Autodesk Fusion 360 part; units mm, degrees
note: some values were not read from the file. Set by a fixed rule: which face or edge a step refers to.
(part 8 of 20)
  spline S44 degree 5 poles (-3.681, 14.0486) (-3.681, 14.0487) (-3.681, 14.0488) (-3.6811, 14.0491) (-3.6812, 14.0494) (-3.6813, 14.0499) (-3.6815, 14.0505) (-3.6817, 14.0512) (-3.6819, 14.0519) (-3.6821, 14.0528) (-3.6824, 14.0537) (-3.6827, 14.0546) (-3.683, 14.0557) (-3.6833, 14.0568) (-3.6837, 14.058) (-3.6841, 14.0592) (-3.6845, 14.0606) (-3.6849, 14.0619) (-3.6853, 14.0634) (-3.6858, 14.0649) (-3.6863, 14.0665) (-3.6869, 14.0682) (-3.6874, 14.0699) (-3.688, 14.0717) (-3.6886, 14.0736) (-3.6892, 14.0755) (-3.6899, 14.0775) (-3.6906, 14.0795) (-3.6913, 14.0816) (-3.692, 14.0838) (-3.6928, 14.086) (-3.6936, 14.0883) (-3.6944, 14.0906) (-3.6952, 14.093) (-3.6961, 14.0955) (-3.697, 14.098) (-3.6979, 14.1006) (-3.6988, 14.1032) (-3.6998, 14.1059) (-3.7008, 14.1086) (-3.7018, 14.1114) (-3.7029, 14.1143) (-3.704, 14.1172) (-3.7051, 14.1202) (-3.7062, 14.1232) (-3.7073, 14.1262) (-3.7085, 14.1293) (-3.7097, 14.1325) (-3.711, 14.1357) (-3.7123, 14.139) (-3.7136, 14.1423) (-3.7149, 14.1457) (-3.7162, 14.1491) (-3.7176, 14.1525) (-3.719, 14.1561) (-3.7204, 14.1596) (-3.7219, 14.1632) (-3.7234, 14.1669) (-3.7249, 14.1706) (-3.7265, 14.1743) (-3.728, 14.1781) (-3.7296, 14.1819) (-3.7313, 14.1858) (-3.7329, 14.1898) (-3.7346, 14.1937) (-3.7363, 14.1977) (-3.7381, 14.2018) (-3.7398, 14.2059) (-3.7416, 14.21) (-3.7435, 14.2142) (-3.7453, 14.2185) (-3.7472, 14.2227) (-3.7491, 14.227) (-3.7511, 14.2314) (-3.753, 14.2358) (-3.755, 14.2402) (-3.7571, 14.2447) (-3.7591, 14.2492) (-3.7612, 14.2537) (-3.7633, 14.2583) (-3.7655, 14.263) (-3.7676, 14.2676) (-3.7698, 14.2723) (-3.7721, 14.2771) (-3.7743, 14.2819) (-3.7766, 14.2867) (-3.7789, 14.2915) (-3.7813, 14.2964) (-3.7836, 14.3013) (-3.7861, 14.3063) (-3.7885, 14.3113) (-3.791, 14.3163) (-3.7934, 14.3214) (-3.796, 14.3265) (-3.7985, 14.3316) (-3.8011, 14.3368) (-3.8037, 14.342) (-3.8063, 14.3473) (-3.809, 14.3525) (-3.8117, 14.3578) (-3.8144, 14.3632) (-3.8172, 14.3685) (-3.82, 14.3739) (-3.8228, 14.3794) (-3.8257, 14.3848) (-3.8285, 14.3903) (-3.8314, 14.3959) (-3.8344, 14.4014) (-3.8373, 14.407) (-3.8403, 14.4126) (-3.8434, 14.4183) (-3.8464, 14.424) (-3.8495, 14.4297) (-3.8526, 14.4354) (-3.8558, 14.4412) (-3.8589, 14.447) (-3.8621, 14.4528) (-3.8654, 14.4587) (-3.8686, 14.4645) (-3.8719, 14.4704) (-3.8752, 14.4764) (-3.8786, 14.4824) (-3.882, 14.4883) (-3.8854, 14.4944) (-3.8888, 14.5004) (-3.8923, 14.5065) (-3.8958, 14.5126) (-3.8993, 14.5187) (-3.9029, 14.5249) (-3.9065, 14.5311) (-3.9101, 14.5373) (-3.9138, 14.5435) (-3.9175, 14.5497) (-3.9212, 14.556) (-3.9249, 14.5623) (-3.9287, 14.5687) (-3.9325, 14.575) (-3.9363, 14.5814) (-3.9402, 14.5878) (-3.9441, 14.5942) (-3.948, 14.6007) (-3.952, 14.6072) (-3.9559, 14.6137) (-3.96, 14.6202) (-3.964, 14.6267) (-3.9681, 14.6333) (-3.9722, 14.6399) (-3.9763, 14.6465) (-3.9805, 14.6531) (-3.9847, 14.6598) (-3.9889, 14.6665) (-3.9932, 14.6731) (-3.9974, 14.6799) (-4.0018, 14.6866) (-4.0061, 14.6934) (-4.0105, 14.7002) (-4.0149, 14.707) (-4.0193, 14.7138) (-4.0238, 14.7206) (-4.0283, 14.7275) (-4.0328, 14.7344) (-4.0374, 14.7413) (-4.042, 14.7482) (-4.0466, 14.7551) (-4.0512, 14.7621) (-4.0559, 14.7691) (-4.0606, 14.7761) (-4.0654, 14.7831) (-4.0701, 14.7901) (-4.0749, 14.7972) (-4.0798, 14.8043) (-4.0846, 14.8114) (-4.0895, 14.8185) (-4.0944, 14.8256) (-4.0994, 14.8328) (-4.1044, 14.8399) (-4.1094, 14.8471) (-4.1144, 14.8543) (-4.1195, 14.8615) (-4.1246, 14.8687) (-4.1297, 14.876) (-4.1349, 14.8833) (-4.1401, 14.8905) (-4.1453, 14.8978) (-4.1506, 14.9052) (-4.1559, 14.9125) (-4.1612, 14.9198) (-4.1665, 14.9272) (-4.1719, 14.9346) (-4.1773, 14.942) (-4.1827, 14.9494) (-4.1882, 14.9568) (-4.1937, 14.9642) (-4.1992, 14.9717) (-4.2048, 14.9791) (-4.2104, 14.9866) (-4.216, 14.9941) (-4.2216, 15.0016) (-4.2273, 15.0092) (-4.233, 15.0167) (-4.2388, 15.0242) (-4.2445, 15.0318) (-4.2503, 15.0394) (-4.2562, 15.047) (-4.262, 15.0546) (-4.2679, 15.0622) (-4.2738, 15.0698) (-4.2798, 15.0775) (-4.2858, 15.0851) (-4.2918, 15.0928) (-4.2978, 15.1005) (-4.3039, 15.1082) (-4.31, 15.1159) (-4.3161, 15.1236) (-4.3223, 15.1313) (-4.3285, 15.1391) (-4.3347, 15.1468) (-4.3409, 15.1546) (-4.3472, 15.1624) (-4.3535, 15.1702) (-4.3599, 15.178) (-4.3662, 15.1858) (-4.3726, 15.1936) (-4.3791, 15.2014) (-4.3855, 15.2093) (-4.392, 15.2171) (-4.3985, 15.225) (-4.4051, 15.2329) (-4.4117, 15.2407) (-4.4183, 15.2486) (-4.4249, 15.2565) (-4.4316, 15.2645) (-4.4383, 15.2724) (-4.445, 15.2803) (-4.4518, 15.2883) (-4.4586, 15.2962) (-4.4654, 15.3042) (-4.4722, 15.3121) (-4.4791, 15.3201) (-4.486, 15.3281) (-4.493, 15.3361) (-4.4985, 15.3425) (-4.5027, 15.3473) (-4.5055, 15.3505) (-4.5069, 15.3521) knots 0 0 0 0 0 0 0.00416667 0.00833333 0.0125 0.01666667 0.02083333 0.025 0.02916667 0.03333333 0.0375 0.04166667 0.04583333 0.05 0.05416667 0.05833333 0.0625 0.06666667 0.07083333 0.075 0.07916667 0.08333333 0.0875 0.09166667 0.09583333 0.1 0.10416667 0.10833333 0.1125 0.11666667 0.12083333 0.125 0.12916667 0.13333333 0.1375 0.14166667 0.14583333 0.15 0.15416667 0.15833333 0.1625 0.16666667 0.17083333 0.175 0.17916667 0.18333333 0.1875 0.19166667 0.19583333 0.2 0.20416667 0.20833333 0.2125 0.21666667 0.22083333 0.225 0.22916667 0.23333333 0.2375 0.24166667 0.24583333 0.25 0.25416667 0.25833333 0.2625 0.26666667 0.27083333 0.275 0.27916667 0.28333333 0.2875 0.29166667 0.29583333 0.3 0.30416667 0.30833333 0.3125 0.31666667 0.32083333 0.325 0.32916667 0.33333333 0.3375 0.34166667 0.34583333 0.35 0.35416667 0.35833333 0.3625 0.36666667 0.37083333 0.375 0.37916667 0.38333333 0.3875 0.39166667 0.39583333 0.4 0.40416667 0.40833333 0.4125 0.41666667 0.42083333 0.425 0.42916667 0.43333333 0.4375 0.44166667 0.44583333 0.45 0.45416667 0.45833333 0.4625 0.46666667 0.47083333 0.475 0.47916667 0.48333333 0.4875 0.49166667 0.49583333 0.5 0.50416667 0.50833333 0.5125 0.51666667 0.52083333 0.525 0.52916667 0.53333333 0.5375 0.54166667 0.54583333 0.55 0.55416667 0.55833333 0.5625 0.56666667 0.57083333 0.575 0.57916667 0.58333333 0.5875 0.59166667 0.59583333 0.6 0.60416667 0.60833333 0.6125 0.61666667 0.62083333 0.625 0.62916667 0.63333333 0.6375 0.64166667 0.64583333 0.65 0.65416667 0.65833333 0.6625 0.66666667 0.67083333 0.675 0.67916667 0.68333333 0.6875 0.69166667 0.69583333 0.7 0.70416667 0.70833333 0.7125 0.71666667 0.72083333 0.725 0.72916667 0.73333333 0.7375 0.74166667 0.74583333 0.75 0.75416667 0.75833333 0.7625 0.76666667 0.77083333 0.775 0.77916667 0.78333333 0.7875 0.79166667 0.79583333 0.8 0.80416667 0.80833333 0.8125 0.81666667 0.82083333 0.825 0.82916667 0.83333333 0.8375 0.84166667 0.84583333 0.85 0.85416667 0.85833333 0.8625 0.86666667 0.87083333 0.875 0.87916667 0.88333333 0.8875 0.89166667 0.89583333 0.9 0.90416667 0.90833333 0.9125 0.91666667 0.92083333 0.925 0.92916667 0.93333333 0.9375 0.94166667 0.94583333 0.95 0.95416667 0.95833333 0.9625 0.96666667 0.97083333 0.975 0.97916667 0.98333333 0.9875 0.99166667 0.99583333 1 1 1 1 1 1
  spline S45 degree 5 poles (-12.6699, -9.771) (-12.6679, -9.7705) (-12.6637, -9.7696) (-12.6575, -9.7682) (-12.6492, -9.7663) (-12.6389, -9.7639) (-12.6286, -9.7615) (-12.6184, -9.7591) (-12.6081, -9.7566) (-12.5979, -9.7542) (-12.5878, -9.7518) (-12.5776, -9.7493) (-12.5675, -9.7469) (-12.5574, -9.7444) (-12.5474, -9.7419) (-12.5374, -9.7394) (-12.5274, -9.7369) (-12.5174, -9.7344) (-12.5075, -9.7319) (-12.4976, -9.7293) (-12.4877, -9.7268) (-12.4779, -9.7243) (-12.4681, -9.7217) (-12.4583, -9.7191) (-12.4486, -9.7166) (-12.4389, -9.714) (-12.4292, -9.7114) (-12.4195, -9.7088) (-12.4099, -9.7062) (-12.4003, -9.7036) (-12.3908, -9.7009) (-12.3812, -9.6983) (-12.3717, -9.6957) (-12.3623, -9.693) (-12.3528, -9.6904) (-12.3434, -9.6877) (-12.3341, -9.685) (-12.3247, -9.6823) (-12.3154, -9.6797) (-12.3062, -9.677) (-12.2969, -9.6743) (-12.2877, -9.6716) (-12.2785, -9.6688) (-12.2694, -9.6661) (-12.2603, -9.6634) (-12.2512, -9.6607) (-12.2421, -9.6579) (-12.2331, -9.6552) (-12.2241, -9.6524) (-12.2152, -9.6496) (-12.2063, -9.6469) (-12.1974, -9.6441) (-12.1885, -9.6413) (-12.1797, -9.6385) (-12.1709, -9.6357) (-12.1622, -9.6329) (-12.1535, -9.6301) (-12.1448, -9.6273) (-12.1361, -9.6245) (-12.1275, -9.6217) (-12.1189, -9.6189) (-12.1104, -9.616) (-12.1018, -9.6132) (-12.0934, -9.6104) (-12.0849, -9.6075) (-12.0765, -9.6047) (-12.0681, -9.6018) (-12.0598, -9.599) (-12.0515, -9.5961) (-12.0432, -9.5933) (-12.035, -9.5904) (-12.0267, -9.5875) (-12.0186, -9.5846) (-12.0104, -9.5818) (-12.0023, -9.5789) (-11.9943, -9.576) (-11.9862, -9.5731) (-11.9782, -9.5702) (-11.9703, -9.5673) (-11.9624, -9.5644) (-11.9545, -9.5615) (-11.9466, -9.5586) (-11.9388, -9.5557) (-11.931, -9.5528) (-11.9233, -9.5499) (-11.9156, -9.547) (-11.9079, -9.5441) (-11.9002, -9.5412) (-11.8926, -9.5383) (-11.8851, -9.5354) (-11.8776, -9.5325) (-11.8701, -9.5295) (-11.8626, -9.5266) (-11.8552, -9.5237) (-11.8478, -9.5208) (-11.8405, -9.5179) (-11.8332, -9.515) (-11.8259, -9.512) (-11.8187, -9.5091) (-11.8115, -9.5062) (-11.8043, -9.5033) (-11.7972, -9.5004) (-11.7901, -9.4975) (-11.7831, -9.4945) (-11.7761, -9.4916) (-11.7691, -9.4887) (-11.7622, -9.4858) (-11.7553, -9.4829) (-11.7484, -9.48) (-11.7416, -9.4771) (-11.7348, -9.4742) (-11.7281, -9.4713) (-11.7214, -9.4684) (-11.7148, -9.4655) (-11.7081, -9.4626) (-11.7016, -9.4597) (-11.695, -9.4568) (-11.6885, -9.4539) (-11.6821, -9.451) (-11.6756, -9.4482) (-11.6693, -9.4453) (-11.6629, -9.4424) (-11.6566, -9.4396) (-11.6504, -9.4367) (-11.6441, -9.4338) (-11.638, -9.431) (-11.6318, -9.4281) (-11.6257, -9.4253) (-11.6197, -9.4225) (-11.6137, -9.4196) (-11.6077, -9.4168) (-11.6017, -9.414) (-11.5959, -9.4112) (-11.59, -9.4084) (-11.5842, -9.4056) (-11.5784, -9.4028) (-11.5727, -9.4) (-11.567, -9.3972) (-11.5614, -9.3944) (-11.5558, -9.3917) (-11.5502, -9.3889) (-11.5447, -9.3862) (-11.5392, -9.3834) (-11.5338, -9.3807) (-11.5284, -9.378) (-11.5231, -9.3753) (-11.5178, -9.3725) (-11.5125, -9.3699) (-11.5073, -9.3672) (-11.5021, -9.3645) (-11.497, -9.3618) (-11.4919, -9.3592) (-11.4869, -9.3565) (-11.4819, -9.3539) (-11.4769, -9.3513) (-11.472, -9.3487) (-11.4672, -9.3461) (-11.4623, -9.3435) (-11.4576, -9.3409) (-11.4528, -9.3383) (-11.4482, -9.3358) (-11.4435, -9.3332) (-11.4389, -9.3307) (-11.4344, -9.3282) (-11.4299, -9.3257) (-11.4254, -9.3232) (-11.421, -9.3207) (-11.4167, -9.3183) (-11.4123, -9.3158) (-11.4081, -9.3134) (-11.4038, -9.311) (-11.3997, -9.3086) (-11.3955, -9.3062) (-11.3915, -9.3039) (-11.3874, -9.3015) (-11.3834, -9.2992) (-11.3795, -9.2969) (-11.3756, -9.2946) (-11.3718, -9.2923) (-11.368, -9.2901) (-11.3642, -9.2878) (-11.3605, -9.2856) (-11.3569, -9.2834) (-11.3533, -9.2812) (-11.3497, -9.2791) (-11.3462, -9.2769) (-11.3428, -9.2748) (-11.3394, -9.2727) (-11.336, -9.2706) (-11.3327, -9.2685) (-11.3295, -9.2665) (-11.3263, -9.2645) (-11.3231, -9.2625) (-11.32, -9.2605) (-11.317, -9.2586) (-11.314, -9.2567) (-11.311, -9.2548) (-11.3081, -9.2529) (-11.3053, -9.2511) (-11.3025, -9.2492) (-11.2998, -9.2474) (-11.2971, -9.2457) (-11.2944, -9.2439) (-11.2919, -9.2422) (-11.2893, -9.2405) (-11.2869, -9.2389) (-11.2844, -9.2372) (-11.2821, -9.2356) (-11.2798, -9.2341) (-11.2775, -9.2325) (-11.2753, -9.231) (-11.2732, -9.2295) (-11.2711, -9.2281) (-11.269, -9.2266) (-11.2671, -9.2253) (-11.2651, -9.2239) (-11.2633, -9.2226) (-11.2615, -9.2213) (-11.2597, -9.22) (-11.258, -9.2188) (-11.2564, -9.2177) (-11.2548, -9.2165) (-11.2533, -9.2154) (-11.2518, -9.2143) (-11.2504, -9.2133) (-11.2491, -9.2123) (-11.2478, -9.2113) (-11.2465, -9.2104) (-11.2454, -9.2096) (-11.2443, -9.2087) (-11.2432, -9.2079) (-11.2422, -9.2072) (-11.2413, -9.2065) (-11.2404, -9.2058) (-11.2396, -9.2052) (-11.2389, -9.2046) (-11.2382, -9.2041) (-11.2376, -9.2036) (-11.2371, -9.2032) (-11.2366, -9.2028) (-11.2362, -9.2025) (-11.2359, -9.2022) (-11.2357, -9.2021) (-11.2356, -9.202) (-11.2355, -9.202) knots -1 -1 -1 -1 -1 -1 -0.99583333 -0.99166667 -0.9875 -0.98333333 -0.97916667 -0.975 -0.97083333 -0.96666667 -0.9625 -0.95833333 -0.95416667 -0.95 -0.94583333 -0.94166667 -0.9375 -0.93333333 -0.92916667 -0.925 -0.92083333 -0.91666667 -0.9125 -0.90833333 -0.90416667 -0.9 -0.89583333 -0.89166667 -0.8875 -0.88333333 -0.87916667 -0.875 -0.87083333 -0.86666667 -0.8625 -0.85833333 -0.85416667 -0.85 -0.84583333 -0.84166667 -0.8375 -0.83333333 -0.82916667 -0.825 -0.82083333 -0.81666667 -0.8125 -0.80833333 -0.80416667 -0.8 -0.79583333 -0.79166667 -0.7875 -0.78333333 -0.77916667 -0.775 -0.77083333 -0.76666667 -0.7625 -0.75833333 -0.75416667 -0.75 -0.74583333 -0.74166667 -0.7375 -0.73333333 -0.72916667 -0.725 -0.72083333 -0.71666667 -0.7125 -0.70833333 -0.70416667 -0.7 -0.69583333 -0.69166667 -0.6875 -0.68333333 -0.67916667 -0.675 -0.67083333 -0.66666667 -0.6625 -0.65833333 -0.65416667 -0.65 -0.64583333 -0.64166667 -0.6375 -0.63333333 -0.62916667 -0.625 -0.62083333 -0.61666667 -0.6125 -0.60833333 -0.60416667 -0.6 -0.59583333 -0.59166667 -0.5875 -0.58333333 -0.57916667 -0.575 -0.57083333 -0.56666667 -0.5625 -0.55833333 -0.55416667 -0.55 -0.54583333 -0.54166667 -0.5375 -0.53333333 -0.52916667 -0.525 -0.52083333 -0.51666667 -0.5125 -0.50833333 -0.50416667 -0.5 -0.49583333 -0.49166667 -0.4875 -0.48333333 -0.47916667 -0.475 -0.47083333 -0.46666667 -0.4625 -0.45833333 -0.45416667 -0.45 -0.44583333 -0.44166667 -0.4375 -0.43333333 -0.42916667 -0.425 -0.42083333 -0.41666667 -0.4125 -0.40833333 -0.40416667 -0.4 -0.39583333 -0.39166667 -0.3875 -0.38333333 -0.37916667 -0.375 -0.37083333 -0.36666667 -0.3625 -0.35833333 -0.35416667 -0.35 -0.34583333 -0.34166667 -0.3375 -0.33333333 -0.32916667 -0.325 -0.32083333 -0.31666667 -0.3125 -0.30833333 -0.30416667 -0.3 -0.29583333 -0.29166667 -0.2875 -0.28333333 -0.27916667 -0.275 -0.27083333 -0.26666667 -0.2625 -0.25833333 -0.25416667 -0.25 -0.24583333 -0.24166667 -0.2375 -0.23333333 -0.22916667 -0.225 -0.22083333 -0.21666667 -0.2125 -0.20833333 -0.20416667 -0.2 -0.19583333 -0.19166667 -0.1875 -0.18333333 -0.17916667 -0.175 -0.17083333 -0.16666667 -0.1625 -0.15833333 -0.15416667 -0.15 -0.14583333 -0.14166667 -0.1375 -0.13333333 -0.12916667 -0.125 -0.12083333 -0.11666667 -0.1125 -0.10833333 -0.10416667 -0.1 -0.09583333 -0.09166667 -0.0875 -0.08333333 -0.07916667 -0.075 -0.07083333 -0.06666667 -0.0625 -0.05833333 -0.05416667 -0.05 -0.04583333 -0.04166667 -0.0375 -0.03333333 -0.02916667 -0.025 -0.02083333 -0.01666667 -0.0125 -0.00833333 -0.00416667 0 0 0 0 0 0
  line L87 (-3.6808, 14.048) -> (-3.681, 14.0486)
  line L88 (-2.3514, 14.3312) -> (-2.3513, 14.3306)
  spline S46 degree 5 poles (-10.326, -10.2121) (-10.326, -10.2122) (-10.3261, -10.2123) (-10.3263, -10.2124) (-10.3266, -10.2127) (-10.3269, -10.2131) (-10.3274, -10.2135) (-10.3279, -10.214) (-10.3284, -10.2146) (-10.329, -10.2152) (-10.3296, -10.2159) (-10.3303, -10.2166) (-10.3311, -10.2174) (-10.3319, -10.2182) (-10.3327, -10.2191) (-10.3336, -10.2201) (-10.3346, -10.2211) (-10.3356, -10.2222) (-10.3366, -10.2233) (-10.3377, -10.2245) (-10.3388, -10.2257) (-10.34, -10.227) (-10.3412, -10.2284) (-10.3425, -10.2298) (-10.3438, -10.2312) (-10.3451, -10.2327) (-10.3465, -10.2343) (-10.3479, -10.2359) (-10.3494, -10.2376) (-10.3509, -10.2393) (-10.3525, -10.241) (-10.354, -10.2429) (-10.3557, -10.2447) (-10.3573, -10.2467) (-10.359, -10.2486) (-10.3608, -10.2507) (-10.3625, -10.2528) (-10.3643, -10.2549) (-10.3662, -10.2571) (-10.368, -10.2593) (-10.37, -10.2616) (-10.3719, -10.2639) (-10.3739, -10.2663) (-10.3759, -10.2688) (-10.3779, -10.2712) (-10.38, -10.2738) (-10.3821, -10.2764) (-10.3842, -10.279) (-10.3864, -10.2817) (-10.3886, -10.2844) (-10.3908, -10.2872) (-10.3931, -10.29) (-10.3954, -10.2929) (-10.3977, -10.2958) (-10.4, -10.2988) (-10.4024, -10.3018) (-10.4048, -10.3049) (-10.4072, -10.308) (-10.4096, -10.3112) (-10.4121, -10.3144) (-10.4146, -10.3176) (-10.4171, -10.3209) (-10.4197, -10.3243) (-10.4222, -10.3277) (-10.4248, -10.3311) (-10.4274, -10.3346) (-10.4301, -10.3382) (-10.4328, -10.3417) (-10.4354, -10.3454) (-10.4382, -10.349) (-10.4409, -10.3528) (-10.4436, -10.3565) (-10.4464, -10.3603) (-10.4492, -10.3642) (-10.452, -10.3681) (-10.4549, -10.3721) (-10.4577, -10.376) (-10.4606, -10.3801) (-10.4635, -10.3842) (-10.4664, -10.3883) (-10.4694, -10.3925) (-10.4723, -10.3967) (-10.4753, -10.4009) (-10.4783, -10.4052) (-10.4813, -10.4096) (-10.4843, -10.414) (-10.4874, -10.4184) (-10.4904, -10.4229) (-10.4935, -10.4274) (-10.4966, -10.432) (-10.4997, -10.4366) (-10.5028, -10.4412) (-10.506, -10.4459) (-10.5091, -10.4507) (-10.5123, -10.4554) (-10.5155, -10.4603) (-10.5187, -10.4651) (-10.5219, -10.47) (-10.5251, -10.475) (-10.5284, -10.48) (-10.5316, -10.485) (-10.5349, -10.4901) (-10.5382, -10.4952) (-10.5415, -10.5003) (-10.5448, -10.5055) (-10.5481, -10.5108) (-10.5515, -10.516) (-10.5548, -10.5214) (-10.5582, -10.5267) (-10.5615, -10.5321) (-10.5649, -10.5376) (-10.5683, -10.5431) (-10.5717, -10.5486) (-10.5751, -10.5542) (-10.5785, -10.5598) (-10.582, -10.5654) (-10.5854, -10.5711) (-10.5889, -10.5768) (-10.5923, -10.5826) (-10.5958, -10.5884) (-10.5993, -10.5943) (-10.6028, -10.6001) (-10.6063, -10.6061) (-10.6098, -10.612) (-10.6133, -10.618) (-10.6168, -10.6241) (-10.6204, -10.6302) (-10.6239, -10.6363) (-10.6275, -10.6425) (-10.631, -10.6487) (-10.6346, -10.6549) (-10.6381, -10.6612) (-10.6417, -10.6675) (-10.6453, -10.6738) (-10.6489, -10.6802) (-10.6525, -10.6867) (-10.6561, -10.6931) (-10.6597, -10.6997) (-10.6633, -10.7062) (-10.6669, -10.7128) (-10.6706, -10.7194) (-10.6742, -10.7261) (-10.6778, -10.7328) (-10.6815, -10.7395) (-10.6851, -10.7463) (-10.6888, -10.7531) (-10.6924, -10.7599) (-10.6961, -10.7668) (-10.6997, -10.7738) (-10.7034, -10.7807) (-10.7071, -10.7877) (-10.7107, -10.7947) (-10.7144, -10.8018) (-10.7181, -10.8089) (-10.7218, -10.8161) (-10.7255, -10.8233) (-10.7292, -10.8305) (-10.7328, -10.8377) (-10.7365, -10.845) (-10.7402, -10.8523) (-10.7439, -10.8597) (-10.7476, -10.8671) (-10.7513, -10.8745) (-10.755, -10.882) (-10.7587, -10.8895) (-10.7625, -10.8971) (-10.7662, -10.9046) (-10.7699, -10.9123) (-10.7736, -10.9199) (-10.7773, -10.9276) (-10.781, -10.9353) (-10.7847, -10.9431) (-10.7884, -10.9509) (-10.7921, -10.9587) (-10.7958, -10.9666) (-10.7996, -10.9745) (-10.8033, -10.9824) (-10.807, -10.9903) (-10.8107, -10.9984) (-10.8144, -11.0064) (-10.8181, -11.0145) (-10.8218, -11.0226) (-10.8255, -11.0307) (-10.8292, -11.0389) (-10.833, -11.0471) (-10.8367, -11.0553) (-10.8404, -11.0636) (-10.8441, -11.0719) (-10.8478, -11.0803) (-10.8515, -11.0886) (-10.8552, -11.097) (-10.8589, -11.1055) (-10.8625, -11.114) (-10.8662, -11.1225) (-10.8699, -11.131) (-10.8736, -11.1396) (-10.8773, -11.1482) (-10.881, -11.1569) (-10.8847, -11.1655) (-10.8883, -11.1743) (-10.892, -11.183) (-10.8957, -11.1918) (-10.8993, -11.2006) (-10.903, -11.2094) (-10.9066, -11.2183) (-10.9103, -11.2272) (-10.9139, -11.2362) (-10.9176, -11.2451) (-10.9212, -11.2541) (-10.9249, -11.2632) (-10.9285, -11.2723) (-10.9321, -11.2814) (-10.9358, -11.2905) (-10.9394, -11.2997) (-10.943, -11.3089) (-10.9466, -11.3181) (-10.9502, -11.3274) (-10.9538, -11.3367) (-10.9574, -11.346) (-10.961, -11.3553) (-10.9646, -11.3647) (-10.9682, -11.3742) (-10.9717, -11.3836) (-10.9753, -11.3931) (-10.9789, -11.4026) (-10.9824, -11.4122) (-10.986, -11.4217) (-10.9895, -11.4313) (-10.993, -11.441) (-10.9966, -11.4507) (-11.0001, -11.4604) (-11.0036, -11.4701) (-11.0071, -11.4799) (-11.0106, -11.4897) (-11.0141, -11.4995) (-11.0176, -11.5093) (-11.0211, -11.5192) (-11.0246, -11.5291) (-11.028, -11.5391) (-11.0315, -11.5491) (-11.035, -11.5591) (-11.0377, -11.5671) (-11.0398, -11.5731) (-11.0412, -11.5772) (-11.0419, -11.5792) knots 0 0 0 0 0 0 0.00416667 0.00833333 0.0125 0.01666667 0.02083333 0.025 0.02916667 0.03333333 0.0375 0.04166667 0.04583333 0.05 0.05416667 0.05833333 0.0625 0.06666667 0.07083333 0.075 0.07916667 0.08333333 0.0875 0.09166667 0.09583333 0.1 0.10416667 0.10833333 0.1125 0.11666667 0.12083333 0.125 0.12916667 0.13333333 0.1375 0.14166667 0.14583333 0.15 0.15416667 0.15833333 0.1625 0.16666667 0.17083333 0.175 0.17916667 0.18333333 0.1875 0.19166667 0.19583333 0.2 0.20416667 0.20833333 0.2125 0.21666667 0.22083333 0.225 0.22916667 0.23333333 0.2375 0.24166667 0.24583333 0.25 0.25416667 0.25833333 0.2625 0.26666667 0.27083333 0.275 0.27916667 0.28333333 0.2875 0.29166667 0.29583333 0.3 0.30416667 0.30833333 0.3125 0.31666667 0.32083333 0.325 0.32916667 0.33333333 0.3375 0.34166667 0.34583333 0.35 0.35416667 0.35833333 0.3625 0.36666667 0.37083333 0.375 0.37916667 0.38333333 0.3875 0.39166667 0.39583333 0.4 0.40416667 0.40833333 0.4125 0.41666667 0.42083333 0.425 0.42916667 0.43333333 0.4375 0.44166667 0.44583333 0.45 0.45416667 0.45833333 0.4625 0.46666667 0.47083333 0.475 0.47916667 0.48333333 0.4875 0.49166667 0.49583333 0.5 0.50416667 0.50833333 0.5125 0.51666667 0.52083333 0.525 0.52916667 0.53333333 0.5375 0.54166667 0.54583333 0.55 0.55416667 0.55833333 0.5625 0.56666667 0.57083333 0.575 0.57916667 0.58333333 0.5875 0.59166667 0.59583333 0.6 0.60416667 0.60833333 0.6125 0.61666667 0.62083333 0.625 0.62916667 0.63333333 0.6375 0.64166667 0.64583333 0.65 0.65416667 0.65833333 0.6625 0.66666667 0.67083333 0.675 0.67916667 0.68333333 0.6875 0.69166667 0.69583333 0.7 0.70416667 0.70833333 0.7125 0.71666667 0.72083333 0.725 0.72916667 0.73333333 0.7375 0.74166667 0.74583333 0.75 0.75416667 0.75833333 0.7625 0.76666667 0.77083333 0.775 0.77916667 0.78333333 0.7875 0.79166667 0.79583333 0.8 0.80416667 0.80833333 0.8125 0.81666667 0.82083333 0.825 0.82916667 0.83333333 0.8375 0.84166667 0.84583333 0.85 0.85416667 0.85833333 0.8625 0.86666667 0.87083333 0.875 0.87916667 0.88333333 0.8875 0.89166667 0.89583333 0.9 0.90416667 0.90833333 0.9125 0.91666667 0.92083333 0.925 0.92916667 0.93333333 0.9375 0.94166667 0.94583333 0.95 0.95416667 0.95833333 0.9625 0.96666667 0.97083333 0.975 0.97916667 0.98333333 0.9875 0.99166667 0.99583333 1 1 1 1 1 1
  arc A54 (-7.5526, 11.49) -> (-8.5938, 10.7336) centre (0, 0) ccw
  line L89 (-6.1743, 12.2858) -> (-6.5211, 12.9757)
  arc A55 (-11.0419, -11.5792) -> (-10.3616, -12.1917) centre (0, 0) ccw
  arc A56 (-10.6376, -8.7123) -> (-9.7765, -9.6687) centre (0, 0) ccw
  line L90 (-9.0764, 11.3364) -> (-9.0768, 11.3369)
  spline S47 degree 5 poles (-5.3776, 15.0692) (-5.3777, 15.0671) (-5.3781, 15.0629) (-5.3787, 15.0565) (-5.3794, 15.0481) (-5.3804, 15.0375) (-5.3813, 15.027) (-5.3821, 15.0165) (-5.383, 15.006) (-5.3838, 14.9956) (-5.3846, 14.9851) (-5.3854, 14.9747) (-5.3862, 14.9644) (-5.387, 14.954) (-5.3877, 14.9437) (-5.3885, 14.9334) (-5.3892, 14.9231) (-5.3899, 14.9129) (-5.3905, 14.9027) (-5.3912, 14.8925) (-5.3918, 14.8823) (-5.3924, 14.8722) (-5.393, 14.862) (-5.3936, 14.852) (-5.3942, 14.8419) (-5.3947, 14.8319) (-5.3953, 14.8218) (-5.3958, 14.8119) (-5.3963, 14.8019) (-5.3967, 14.792) (-5.3972, 14.7821) (-5.3976, 14.7722) (-5.3981, 14.7624) (-5.3985, 14.7525) (-5.3988, 14.7427) (-5.3992, 14.733) (-5.3996, 14.7232) (-5.3999, 14.7135) (-5.4002, 14.7038) (-5.4005, 14.6942) (-5.4008, 14.6846) (-5.4011, 14.675) (-5.4013, 14.6654) (-5.4016, 14.6559) (-5.4018, 14.6464) (-5.402, 14.6369) (-5.4022, 14.6274) (-5.4024, 14.618) (-5.4025, 14.6086) (-5.4027, 14.5992) (-5.4028, 14.5899) (-5.4029, 14.5806) (-5.403, 14.5713) (-5.4031, 14.5621) (-5.4031, 14.5528) (-5.4032, 14.5437) (-5.4032, 14.5345) (-5.4032, 14.5254) (-5.4032, 14.5163) (-5.4032, 14.5072) (-5.4031, 14.4982) (-5.4031, 14.4892) (-5.403, 14.4802) (-5.403, 14.4712) (-5.4029, 14.4623) (-5.4028, 14.4535) (-5.4026, 14.4446) (-5.4025, 14.4358) (-5.4023, 14.427) (-5.4022, 14.4182) (-5.402, 14.4095) (-5.4018, 14.4008) (-5.4016, 14.3922) (-5.4014, 14.3835) (-5.4011, 14.3749) (-5.4009, 14.3664) (-5.4006, 14.3578) (-5.4003, 14.3493) (-5.4001, 14.3409) (-5.3998, 14.3325) (-5.3994, 14.3241) (-5.3991, 14.3157) (-5.3988, 14.3074) (-5.3984, 14.2991) (-5.398, 14.2908) (-5.3976, 14.2826) (-5.3973, 14.2744) (-5.3968, 14.2662) (-5.3964, 14.2581) (-5.396, 14.25) (-5.3955, 14.2419) (-5.3951, 14.2339) (-5.3946, 14.2259) (-5.3941, 14.2179) (-5.3936, 14.21) (-5.3931, 14.2021) (-5.3926, 14.1943) (-5.3921, 14.1865) (-5.3915, 14.1787) (-5.391, 14.171) (-5.3904, 14.1632) (-5.3899, 14.1556) (-5.3893, 14.1479) (-5.3887, 14.1403) (-5.3881, 14.1328) (-5.3874, 14.1253) (-5.3868, 14.1178) (-5.3862, 14.1103) (-5.3855, 14.1029) (-5.3849, 14.0955) (-5.3842, 14.0882) (-5.3835, 14.0809) (-5.3828, 14.0736) (-5.3821, 14.0664) (-5.3814, 14.0592) (-5.3807, 14.0521) (-5.38, 14.0449) (-5.3793, 14.0379) (-5.3785, 14.0308) (-5.3778, 14.0238) (-5.377, 14.0169) (-5.3762, 14.01) (-5.3755, 14.0031) (-5.3747, 13.9963) (-5.3739, 13.9895) (-5.3731, 13.9827) (-5.3723, 13.976) (-5.3714, 13.9693) (-5.3706, 13.9627) (-5.3698, 13.9561) (-5.3689, 13.9495) (-5.3681, 13.943) (-5.3672, 13.9365) (-5.3664, 13.9301) (-5.3655, 13.9237) (-5.3646, 13.9173) (-5.3638, 13.911) (-5.3629, 13.9048) (-5.362, 13.8986) (-5.3611, 13.8924) (-5.3602, 13.8862) (-5.3593, 13.8801) (-5.3583, 13.8741) (-5.3574, 13.8681) (-5.3565, 13.8621) (-5.3556, 13.8562) (-5.3546, 13.8503) (-5.3537, 13.8445) (-5.3528, 13.8387) (-5.3518, 13.833) (-5.3509, 13.8273) (-5.3499, 13.8216) (-5.3489, 13.816) (-5.348, 13.8104) (-5.347, 13.8049) (-5.3461, 13.7994) (-5.3451, 13.794) (-5.3441, 13.7886) (-5.3431, 13.7833) (-5.3422, 13.778) (-5.3412, 13.7728) (-5.3402, 13.7676) (-5.3392, 13.7624) (-5.3382, 13.7573) (-5.3372, 13.7523) (-5.3363, 13.7473) (-5.3353, 13.7423) (-5.3343, 13.7374) (-5.3333, 13.7325) (-5.3323, 13.7277) (-5.3313, 13.723) (-5.3303, 13.7183) (-5.3293, 13.7136) (-5.3284, 13.709) (-5.3274, 13.7044) (-5.3264, 13.6999) (-5.3254, 13.6954) (-5.3244, 13.691) (-5.3235, 13.6867) (-5.3225, 13.6824) (-5.3215, 13.6781) (-5.3205, 13.6739) (-5.3196, 13.6698) (-5.3186, 13.6657) (-5.3176, 13.6616) (-5.3167, 13.6576) (-5.3157, 13.6537) (-5.3148, 13.6498) (-5.3138, 13.646) (-5.3129, 13.6422) (-5.312, 13.6385) (-5.3111, 13.6348) (-5.3101, 13.6312) (-5.3092, 13.6276) (-5.3083, 13.6241) (-5.3074, 13.6207) (-5.3065, 13.6173) (-5.3056, 13.614) (-5.3047, 13.6107) (-5.3039, 13.6075) (-5.303, 13.6043) (-5.3022, 13.6012) (-5.3013, 13.5982) (-5.3005, 13.5952) (-5.2997, 13.5923) (-5.2988, 13.5894) (-5.298, 13.5866) (-5.2972, 13.5839) (-5.2965, 13.5812) (-5.2957, 13.5786) (-5.2949, 13.576) (-5.2942, 13.5735) (-5.2935, 13.5711) (-5.2927, 13.5687) (-5.292, 13.5664) (-5.2913, 13.5641) (-5.2907, 13.5619) (-5.29, 13.5598) (-5.2893, 13.5578) (-5.2887, 13.5558) (-5.2881, 13.5539) (-5.2875, 13.552) (-5.2869, 13.5502) (-5.2863, 13.5485) (-5.2858, 13.5468) (-5.2853, 13.5452) (-5.2848, 13.5437) (-5.2843, 13.5423) (-5.2838, 13.5409) (-5.2833, 13.5396) (-5.2829, 13.5383) (-5.2825, 13.5372) (-5.2821, 13.5361) (-5.2818, 13.5351) (-5.2814, 13.5341) (-5.2811, 13.5332) (-5.2808, 13.5324) (-5.2805, 13.5317) (-5.2803, 13.531) (-5.2801, 13.5305) (-5.2799, 13.53) (-5.2798, 13.5296) (-5.2797, 13.5294) (-5.2796, 13.5293) (-5.2796, 13.5292) knots -1 -1 -1 -1 -1 -1 -0.99583333 -0.99166667 -0.9875 -0.98333333 -0.97916667 -0.975 -0.97083333 -0.96666667 -0.9625 -0.95833333 -0.95416667 -0.95 -0.94583333 -0.94166667 -0.9375 -0.93333333 -0.92916667 -0.925 -0.92083333 -0.91666667 -0.9125 -0.90833333 -0.90416667 -0.9 -0.89583333 -0.89166667 -0.8875 -0.88333333 -0.87916667 -0.875 -0.87083333 -0.86666667 -0.8625 -0.85833333 -0.85416667 -0.85 -0.84583333 -0.84166667 -0.8375 -0.83333333 -0.82916667 -0.825 -0.82083333 -0.81666667 -0.8125 -0.80833333 -0.80416667 -0.8 -0.79583333 -0.79166667 -0.7875 -0.78333333 -0.77916667 -0.775 -0.77083333 -0.76666667 -0.7625 -0.75833333 -0.75416667 -0.75 -0.74583333 -0.74166667 -0.7375 -0.73333333 -0.72916667 -0.725 -0.72083333 -0.71666667 -0.7125 -0.70833333 -0.70416667 -0.7 -0.69583333 -0.69166667 -0.6875 -0.68333333 -0.67916667 -0.675 -0.67083333 -0.66666667 -0.6625 -0.65833333 -0.65416667 -0.65 -0.64583333 -0.64166667 -0.6375 -0.63333333 -0.62916667 -0.625 -0.62083333 -0.61666667 -0.6125 -0.60833333 -0.60416667 -0.6 -0.59583333 -0.59166667 -0.5875 -0.58333333 -0.57916667 -0.575 -0.57083333 -0.56666667 -0.5625 -0.55833333 -0.55416667 -0.55 -0.54583333 -0.54166667 -0.5375 -0.53333333 -0.52916667 -0.525 -0.52083333 -0.51666667 -0.5125 -0.50833333 -0.50416667 -0.5 -0.49583333 -0.49166667 -0.4875 -0.48333333 -0.47916667 -0.475 -0.47083333 -0.46666667 -0.4625 -0.45833333 -0.45416667 -0.45 -0.44583333 -0.44166667 -0.4375 -0.43333333 -0.42916667 -0.425 -0.42083333 -0.41666667 -0.4125 -0.40833333 -0.40416667 -0.4 -0.39583333 -0.39166667 -0.3875 -0.38333333 -0.37916667 -0.375 -0.37083333 -0.36666667 -0.3625 -0.35833333 -0.35416667 -0.35 -0.34583333 -0.34166667 -0.3375 -0.33333333 -0.32916667 -0.325 -0.32083333 -0.31666667 -0.3125 -0.30833333 -0.30416667 -0.3 -0.29583333 -0.29166667 -0.2875 -0.28333333 -0.27916667 -0.275 -0.27083333 -0.26666667 -0.2625 -0.25833333 -0.25416667 -0.25 -0.24583333 -0.24166667 -0.2375 -0.23333333 -0.22916667 -0.225 -0.22083333 -0.21666667 -0.2125 -0.20833333 -0.20416667 -0.2 -0.19583333 -0.19166667 -0.1875 -0.18333333 -0.17916667 -0.175 -0.17083333 -0.16666667 -0.1625 -0.15833333 -0.15416667 -0.15 -0.14583333 -0.14166667 -0.1375 -0.13333333 -0.12916667 -0.125 -0.12083333 -0.11666667 -0.1125 -0.10833333 -0.10416667 -0.1 -0.09583333 -0.09166667 -0.0875 -0.08333333 -0.07916667 -0.075 -0.07083333 -0.06666667 -0.0625 -0.05833333 -0.05416667 -0.05 -0.04583333 -0.04166667 -0.0375 -0.03333333 -0.02916667 -0.025 -0.02083333 -0.01666667 -0.0125 -0.00833333 -0.00416667 0 0 0 0 0 0
  spline S48 degree 5 poles (-12.2236, -7.8421) (-12.2236, -7.8421) (-12.2237, -7.8422) (-12.2239, -7.8423) (-12.2242, -7.8425) (-12.2247, -7.8428) (-12.2252, -7.8431) (-12.2258, -7.8435) (-12.2264, -7.844) (-12.2271, -7.8445) (-12.2279, -7.845) (-12.2287, -7.8455) (-12.2296, -7.8462) (-12.2306, -7.8468) (-12.2316, -7.8475) (-12.2327, -7.8483) (-12.2338, -7.8491) (-12.235, -7.8499) (-12.2363, -7.8508) (-12.2376, -7.8517) (-12.2389, -7.8527) (-12.2403, -7.8537) (-12.2418, -7.8548) (-12.2433, -7.8559) (-12.2449, -7.857) (-12.2465, -7.8582) (-12.2482, -7.8595) (-12.25, -7.8608) (-12.2517, -7.8621) (-12.2536, -7.8634) (-12.2555, -7.8649) (-12.2574, -7.8663) (-12.2594, -7.8678) (-12.2614, -7.8693) (-12.2635, -7.8709) (-12.2656, -7.8726) (-12.2677, -7.8742) (-12.27, -7.8759) (-12.2722, -7.8777) (-12.2745, -7.8795) (-12.2769, -7.8813) (-12.2792, -7.8832) (-12.2817, -7.8851) (-12.2841, -7.8871) (-12.2867, -7.8891) (-12.2892, -7.8911) (-12.2918, -7.8932) (-12.2944, -7.8954) (-12.2971, -7.8975) (-12.2998, -7.8998) (-12.3026, -7.902) (-12.3054, -7.9043) (-12.3082, -7.9066) (-12.3111, -7.909) (-12.314, -7.9115) (-12.3169, -7.9139) (-12.3199, -7.9164) (-12.3229, -7.919) (-12.326, -7.9216) (-12.329, -7.9242) (-12.3322, -7.9268) (-12.3353, -7.9296) (-12.3385, -7.9323) (-12.3417, -7.9351) (-12.345, -7.9379) (-12.3483, -7.9408) (-12.3516, -7.9437) (-12.3549, -7.9467) (-12.3583, -7.9496) (-12.3617, -7.9527) (-12.3652, -7.9558) (-12.3687, -7.9589) (-12.3722, -7.962) (-12.3757, -7.9652) (-12.3793, -7.9684) (-12.3829, -7.9717) (-12.3865, -7.975) (-12.3902, -7.9784) (-12.3938, -7.9818) (-12.3976, -7.9852) (-12.4013, -7.9887) (-12.4051, -7.9922) (-12.4089, -7.9957) (-12.4127, -7.9993) (-12.4165, -8.0029) (-12.4204, -8.0066) (-12.4243, -8.0103) (-12.4282, -8.014) (-12.4322, -8.0178) (-12.4361, -8.0216) (-12.4401, -8.0255) (-12.4442, -8.0294) (-12.4482, -8.0333) (-12.4523, -8.0373) (-12.4564, -8.0413) (-12.4605, -8.0454) (-12.4647, -8.0495) (-12.4688, -8.0536) (-12.473, -8.0578) (-12.4772, -8.062) (-12.4815, -8.0662) (-12.4857, -8.0705) (-12.49, -8.0748) (-12.4943, -8.0792) (-12.4986, -8.0836) (-12.5029, -8.088) (-12.5073, -8.0925) (-12.5117, -8.097) (-12.5161, -8.1015) (-12.5205, -8.1061) (-12.5249, -8.1107) (-12.5294, -8.1154) (-12.5339, -8.1201) (-12.5384, -8.1248) (-12.5429, -8.1296) (-12.5474, -8.1344) (-12.552, -8.1393) (-12.5565, -8.1441) (-12.5611, -8.1491) (-12.5657, -8.154) (-12.5703, -8.159) (-12.575, -8.1641) (-12.5796, -8.1691) (-12.5843, -8.1742) (-12.589, -8.1794) (-12.5937, -8.1846) (-12.5984, -8.1898) (-12.6032, -8.195) (-12.6079, -8.2003) (-12.6127, -8.2056) (-12.6175, -8.211) (-12.6223, -8.2164) (-12.6271, -8.2218) (-12.6319, -8.2273) (-12.6367, -8.2328) (-12.6416, -8.2384) (-12.6465, -8.2439) (-12.6513, -8.2496) (-12.6562, -8.2552) (-12.6612, -8.2609) (-12.6661, -8.2666) (-12.671, -8.2724) (-12.676, -8.2782) (-12.6809, -8.284) (-12.6859, -8.2899) (-12.6909, -8.2958) (-12.6959, -8.3017) (-12.7009, -8.3077) (-12.7059, -8.3137) (-12.7109, -8.3198) (-12.716, -8.3259) (-12.721, -8.332) (-12.7261, -8.3381) (-12.7312, -8.3443) (-12.7363, -8.3505) (-12.7414, -8.3568) (-12.7465, -8.3631) (-12.7516, -8.3694) (-12.7567, -8.3758) (-12.7619, -8.3822) (-12.767, -8.3886) (-12.7722, -8.3951) (-12.7773, -8.4016) (-12.7825, -8.4081) (-12.7877, -8.4147) (-12.7929, -8.4213) (-12.7981, -8.4279) (-12.8033, -8.4346) (-12.8085, -8.4413) (-12.8138, -8.4481) (-12.819, -8.4549) (-12.8242, -8.4617) (-12.8295, -8.4685) (-12.8347, -8.4754) (-12.84, -8.4823) (-12.8453, -8.4893) (-12.8506, -8.4963) (-12.8558, -8.5033) (-12.8611, -8.5103) (-12.8664, -8.5174) (-12.8718, -8.5246) (-12.8771, -8.5317) (-12.8824, -8.5389) (-12.8877, -8.5461) (-12.893, -8.5534) (-12.8984, -8.5607) (-12.9037, -8.568) (-12.9091, -8.5754) (-12.9144, -8.5827) (-12.9198, -8.5902) (-12.9252, -8.5976) (-12.9305, -8.6051) (-12.9359, -8.6126) (-12.9413, -8.6202) (-12.9467, -8.6278) (-12.9521, -8.6354) (-12.9574, -8.6431) (-12.9628, -8.6508) (-12.9682, -8.6585) (-12.9736, -8.6663) (-12.9791, -8.6741) (-12.9845, -8.6819) (-12.9899, -8.6897) (-12.9953, -8.6976) (-13.0007, -8.7055) (-13.0062, -8.7135) (-13.0116, -8.7215) (-13.017, -8.7295) (-13.0224, -8.7376) (-13.0279, -8.7456) (-13.0333, -8.7538) (-13.0388, -8.7619) (-13.0442, -8.7701) (-13.0497, -8.7783) (-13.0551, -8.7866) (-13.0606, -8.7948) (-13.066, -8.8032) (-13.0715, -8.8115) (-13.0769, -8.8199) (-13.0824, -8.8283) (-13.0878, -8.8367) (-13.0933, -8.8452) (-13.0988, -8.8537) (-13.1042, -8.8622) (-13.1097, -8.8708) (-13.1151, -8.8794) (-13.1206, -8.888) (-13.1261, -8.8967) (-13.1315, -8.9054) (-13.137, -8.9141) (-13.1425, -8.9229) (-13.1479, -8.9317) (-13.1534, -8.9405) (-13.1589, -8.9493) (-13.1643, -8.9582) (-13.1698, -8.9671) (-13.1752, -8.9761) (-13.1807, -8.9851) (-13.1862, -8.9941) (-13.1916, -9.0031) (-13.1971, -9.0122) (-13.2015, -9.0195) (-13.2047, -9.0249) (-13.2069, -9.0286) (-13.208, -9.0304) knots 0 0 0 0 0 0 0.00416667 0.00833333 0.0125 0.01666667 0.02083333 0.025 0.02916667 0.03333333 0.0375 0.04166667 0.04583333 0.05 0.05416667 0.05833333 0.0625 0.06666667 0.07083333 0.075 0.07916667 0.08333333 0.0875 0.09166667 0.09583333 0.1 0.10416667 0.10833333 0.1125 0.11666667 0.12083333 0.125 0.12916667 0.13333333 0.1375 0.14166667 0.14583333 0.15 0.15416667 0.15833333 0.1625 0.16666667 0.17083333 0.175 0.17916667 0.18333333 0.1875 0.19166667 0.19583333 0.2 0.20416667 0.20833333 0.2125 0.21666667 0.22083333 0.225 0.22916667 0.23333333 0.2375 0.24166667 0.24583333 0.25 0.25416667 0.25833333 0.2625 0.26666667 0.27083333 0.275 0.27916667 0.28333333 0.2875 0.29166667 0.29583333 0.3 0.30416667 0.30833333 0.3125 0.31666667 0.32083333 0.325 0.32916667 0.33333333 0.3375 0.34166667 0.34583333 0.35 0.35416667 0.35833333 0.3625 0.36666667 0.37083333 0.375 0.37916667 0.38333333 0.3875 0.39166667 0.39583333 0.4 0.40416667 0.40833333 0.4125 0.41666667 0.42083333 0.425 0.42916667 0.43333333 0.4375 0.44166667 0.44583333 0.45 0.45416667 0.45833333 0.4625 0.46666667 0.47083333 0.475 0.47916667 0.48333333 0.4875 0.49166667 0.49583333 0.5 0.50416667 0.50833333 0.5125 0.51666667 0.52083333 0.525 0.52916667 0.53333333 0.5375 0.54166667 0.54583333 0.55 0.55416667 0.55833333 0.5625 0.56666667 0.57083333 0.575 0.57916667 0.58333333 0.5875 0.59166667 0.59583333 0.6 0.60416667 0.60833333 0.6125 0.61666667 0.62083333 0.625 0.62916667 0.63333333 0.6375 0.64166667 0.64583333 0.65 0.65416667 0.65833333 0.6625 0.66666667 0.67083333 0.675 0.67916667 0.68333333 0.6875 0.69166667 0.69583333 0.7 0.70416667 0.70833333 0.7125 0.71666667 0.72083333 0.725 0.72916667 0.73333333 0.7375 0.74166667 0.74583333 0.75 0.75416667 0.75833333 0.7625 0.76666667 0.77083333 0.775 0.77916667 0.78333333 0.7875 0.79166667 0.79583333 0.8 0.80416667 0.80833333 0.8125 0.81666667 0.82083333 0.825 0.82916667 0.83333333 0.8375 0.84166667 0.84583333 0.85 0.85416667 0.85833333 0.8625 0.86666667 0.87083333 0.875 0.87916667 0.88333333 0.8875 0.89166667 0.89583333 0.9 0.90416667 0.90833333 0.9125 0.91666667 0.92083333 0.925 0.92916667 0.93333333 0.9375 0.94166667 0.94583333 0.95 0.95416667 0.95833333 0.9625 0.96666667 0.97083333 0.975 0.97916667 0.98333333 0.9875 0.99166667 0.99583333 1 1 1 1 1 1
  line L91 (-0.6435, 13.7349) -> (-0.6796, 14.5063)
  arc A57 (-8.3931, -13.6219) -> (-7.6003, -14.0796) centre (0, 0) ccw
  arc A58 (-8.5938, -10.7336) -> (-7.5526, -11.49) centre (0, 0) ccw
  spline S49 degree 5 poles (-14.7969, 6.087) (-14.7955, 6.0854) (-14.7926, 6.0823) (-14.7882, 6.0776) (-14.7824, 6.0714) (-14.7752, 6.0637) (-14.768, 6.056) (-14.7608, 6.0483) (-14.7536, 6.0406) (-14.7464, 6.033) (-14.7392, 6.0254) (-14.732, 6.0179) (-14.7248, 6.0104) (-14.7176, 6.0029) (-14.7104, 5.9954) (-14.7033, 5.988) (-14.6961, 5.9806) (-14.689, 5.9732) (-14.6818, 5.9659) (-14.6747, 5.9586) (-14.6675, 5.9513) (-14.6604, 5.9441) (-14.6533, 5.9368) (-14.6462, 5.9297) (-14.6391, 5.9225) (-14.632, 5.9154) (-14.6249, 5.9083) (-14.6178, 5.9012) (-14.6108, 5.8942) (-14.6037, 5.8872) (-14.5966, 5.8802) (-14.5896, 5.8733) (-14.5826, 5.8664) (-14.5755, 5.8595) (-14.5685, 5.8527) (-14.5615, 5.8459) (-14.5545, 5.8391) (-14.5475, 5.8324) (-14.5405, 5.8256) (-14.5336, 5.819) (-14.5266, 5.8123) (-14.5197, 5.8057) (-14.5127, 5.7991) (-14.5058, 5.7925) (-14.4989, 5.786) (-14.492, 5.7795) (-14.4851, 5.773) (-14.4782, 5.7666) (-14.4713, 5.7602) (-14.4644, 5.7538) (-14.4576, 5.7475) (-14.4507, 5.7412) (-14.4439, 5.7349) (-14.4371, 5.7287) (-14.4303, 5.7225) (-14.4235, 5.7163) (-14.4167, 5.7101) (-14.4099, 5.704) (-14.4031, 5.6979) (-14.3964, 5.6919) (-14.3896, 5.6859) (-14.3829, 5.6799) (-14.3762, 5.6739) (-14.3695, 5.668) (-14.3628, 5.6621) (-14.3562, 5.6562) (-14.3495, 5.6504) (-14.3429, 5.6446) (-14.3362, 5.6388) (-14.3296, 5.6331) (-14.323, 5.6274) (-14.3164, 5.6217) (-14.3098, 5.6161) (-14.3033, 5.6105) (-14.2967, 5.6049) (-14.2902, 5.5993) (-14.2837, 5.5938) (-14.2772, 5.5883) (-14.2707, 5.5829) (-14.2642, 5.5775) (-14.2578, 5.5721) (-14.2513, 5.5667) (-14.2449, 5.5614) (-14.2385, 5.5561) (-14.2321, 5.5509) (-14.2257, 5.5457) (-14.2194, 5.5405) (-14.213, 5.5353) (-14.2067, 5.5302) (-14.2004, 5.5251) (-14.1941, 5.52) (-14.1879, 5.515) (-14.1816, 5.51) (-14.1754, 5.505) (-14.1692, 5.5001) (-14.163, 5.4952) (-14.1568, 5.4903) (-14.1506, 5.4855) (-14.1445, 5.4807) (-14.1383, 5.4759) (-14.1322, 5.4712) (-14.1262, 5.4665) (-14.1201, 5.4618) (-14.114, 5.4572) (-14.108, 5.4526) (-14.102, 5.448) (-14.096, 5.4434) (-14.0901, 5.4389) (-14.0841, 5.4344) (-14.0782, 5.43) (-14.0723, 5.4256) (-14.0664, 5.4212) (-14.0606, 5.4169) (-14.0547, 5.4125) (-14.0489, 5.4083) (-14.0431, 5.404) (-14.0373, 5.3998) (-14.0316, 5.3956) (-14.0259, 5.3914) (-14.0202, 5.3873) (-14.0145, 5.3832) (-14.0088, 5.3792) (-14.0032, 5.3752) (-13.9976, 5.3712) (-13.992, 5.3672) (-13.9865, 5.3633) (-13.9809, 5.3594) (-13.9754, 5.3555) (-13.9699, 5.3517) (-13.9645, 5.3479) (-13.959, 5.3441) (-13.9536, 5.3404) (-13.9482, 5.3367) (-13.9429, 5.3331) (-13.9376, 5.3294) (-13.9322, 5.3258) (-13.927, 5.3223) (-13.9217, 5.3187) (-13.9165, 5.3152) (-13.9113, 5.3118) (-13.9061, 5.3083) (-13.901, 5.3049) (-13.8959, 5.3015) (-13.8908, 5.2982) (-13.8858, 5.2949) (-13.8807, 5.2916) (-13.8757, 5.2884) (-13.8708, 5.2852) (-13.8658, 5.282) (-13.8609, 5.2789) (-13.8561, 5.2758) (-13.8512, 5.2727) (-13.8464, 5.2697) (-13.8416, 5.2666) (-13.8369, 5.2637) (-13.8322, 5.2607) (-13.8275, 5.2578) (-13.8228, 5.2549) (-13.8182, 5.2521) (-13.8136, 5.2493) (-13.8091, 5.2465) (-13.8046, 5.2438) (-13.8001, 5.241) (-13.7956, 5.2384) (-13.7912, 5.2357) (-13.7869, 5.2331) (-13.7825, 5.2305) (-13.7782, 5.228) (-13.7739, 5.2254) (-13.7697, 5.223) (-13.7655, 5.2205) (-13.7613, 5.2181) (-13.7572, 5.2157) (-13.7531, 5.2134) (-13.7491, 5.211) (-13.7451, 5.2087) (-13.7411, 5.2065) (-13.7372, 5.2043) (-13.7333, 5.2021) (-13.7294, 5.1999) (-13.7256, 5.1978) (-13.7218, 5.1957) (-13.7181, 5.1936) (-13.7144, 5.1916) (-13.7108, 5.1896) (-13.7072, 5.1877) (-13.7036, 5.1857) (-13.7001, 5.1838) (-13.6966, 5.182) (-13.6932, 5.1801) (-13.6898, 5.1783) (-13.6864, 5.1766) (-13.6831, 5.1749) (-13.6799, 5.1732) (-13.6767, 5.1715) (-13.6735, 5.1698) (-13.6704, 5.1682) (-13.6673, 5.1667) (-13.6643, 5.1651) (-13.6613, 5.1636) (-13.6584, 5.1622) (-13.6555, 5.1607) (-13.6527, 5.1593) (-13.6499, 5.1579) (-13.6472, 5.1566) (-13.6445, 5.1553) (-13.6419, 5.154) (-13.6393, 5.1528) (-13.6368, 5.1515) (-13.6343, 5.1504) (-13.6319, 5.1492) (-13.6296, 5.1481) (-13.6273, 5.147) (-13.625, 5.146) (-13.6228, 5.1449) (-13.6207, 5.1439) (-13.6186, 5.143) (-13.6166, 5.1421) (-13.6147, 5.1412) (-13.6128, 5.1403) (-13.6109, 5.1395) (-13.6091, 5.1387) (-13.6074, 5.1379) (-13.6057, 5.1372) (-13.6042, 5.1365) (-13.6026, 5.1358) (-13.6011, 5.1352) (-13.5997, 5.1346) (-13.5984, 5.134) (-13.5971, 5.1335) (-13.5959, 5.1329) (-13.5948, 5.1325) (-13.5937, 5.132) (-13.5927, 5.1316) (-13.5918, 5.1312) (-13.5909, 5.1309) (-13.5901, 5.1305) (-13.5894, 5.1303) (-13.5887, 5.13) (-13.5882, 5.1298) (-13.5877, 5.1296) (-13.5873, 5.1294) (-13.5871, 5.1293) (-13.587, 5.1293) (-13.5869, 5.1293) knots -1 -1 -1 -1 -1 -1 -0.99583333 -0.99166667 -0.9875 -0.98333333 -0.97916667 -0.975 -0.97083333 -0.96666667 -0.9625 -0.95833333 -0.95416667 -0.95 -0.94583333 -0.94166667 -0.9375 -0.93333333 -0.92916667 -0.925 -0.92083333 -0.91666667 -0.9125 -0.90833333 -0.90416667 -0.9 -0.89583333 -0.89166667 -0.8875 -0.88333333 -0.87916667 -0.875 -0.87083333 -0.86666667 -0.8625 -0.85833333 -0.85416667 -0.85 -0.84583333 -0.84166667 -0.8375 -0.83333333 -0.82916667 -0.825 -0.82083333 -0.81666667 -0.8125 -0.80833333 -0.80416667 -0.8 -0.79583333 -0.79166667 -0.7875 -0.78333333 -0.77916667 -0.775 -0.77083333 -0.76666667 -0.7625 -0.75833333 -0.75416667 -0.75 -0.74583333 -0.74166667 -0.7375 -0.73333333 -0.72916667 -0.725 -0.72083333 -0.71666667 -0.7125 -0.70833333 -0.70416667 -0.7 -0.69583333 -0.69166667 -0.6875 -0.68333333 -0.67916667 -0.675 -0.67083333 -0.66666667 -0.6625 -0.65833333 -0.65416667 -0.65 -0.64583333 -0.64166667 -0.6375 -0.63333333 -0.62916667 -0.625 -0.62083333 -0.61666667 -0.6125 -0.60833333 -0.60416667 -0.6 -0.59583333 -0.59166667 -0.5875 -0.58333333 -0.57916667 -0.575 -0.57083333 -0.56666667 -0.5625 -0.55833333 -0.55416667 -0.55 -0.54583333 -0.54166667 -0.5375 -0.53333333 -0.52916667 -0.525 -0.52083333 -0.51666667 -0.5125 -0.50833333 -0.50416667 -0.5 -0.49583333 -0.49166667 -0.4875 -0.48333333 -0.47916667 -0.475 -0.47083333 -0.46666667 -0.4625 -0.45833333 -0.45416667 -0.45 -0.44583333 -0.44166667 -0.4375 -0.43333333 -0.42916667 -0.425 -0.42083333 -0.41666667 -0.4125 -0.40833333 -0.40416667 -0.4 -0.39583333 -0.39166667 -0.3875 -0.38333333 -0.37916667 -0.375 -0.37083333 -0.36666667 -0.3625 -0.35833333 -0.35416667 -0.35 -0.34583333 -0.34166667 -0.3375 -0.33333333 -0.32916667 -0.325 -0.32083333 -0.31666667 -0.3125 -0.30833333 -0.30416667 -0.3 -0.29583333 -0.29166667 -0.2875 -0.28333333 -0.27916667 -0.275 -0.27083333 -0.26666667 -0.2625 -0.25833333 -0.25416667 -0.25 -0.24583333 -0.24166667 -0.2375 -0.23333333 -0.22916667 -0.225 -0.22083333 -0.21666667 -0.2125 -0.20833333 -0.20416667 -0.2 -0.19583333 -0.19166667 -0.1875 -0.18333333 -0.17916667 -0.175 -0.17083333 -0.16666667 -0.1625 -0.15833333 -0.15416667 -0.15 -0.14583333 -0.14166667 -0.1375 -0.13333333 -0.12916667 -0.125 -0.12083333 -0.11666667 -0.1125 -0.10833333 -0.10416667 -0.1 -0.09583333 -0.09166667 -0.0875 -0.08333333 -0.07916667 -0.075 -0.07083333 -0.06666667 -0.0625 -0.05833333 -0.05416667 -0.05 -0.04583333 -0.04166667 -0.0375 -0.03333333 -0.02916667 -0.025 -0.02083333 -0.01666667 -0.0125 -0.00833333 -0.00416667 0 0 0 0 0 0
  line L92 (-8.5938, 10.7336) -> (-9.0764, 11.3364)